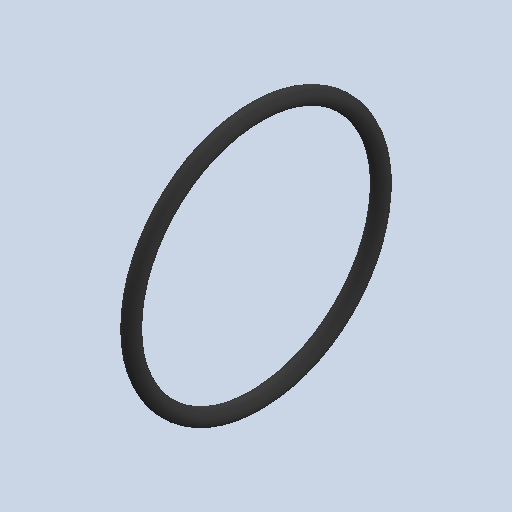
# Autodesk Inventor part: RD013_オーリング
Saved by Autodesk Inventor 2022 (Build 260153000, 153)
## iProperties
Created: 2021-10-14
Part Number: RD013_オーリング
Material: ゴム
Document SubType Name: Modeling
Designer: gilte
Density: 0.93 g/cm^3
Appearance: ゴム - 黒
Author: gilte
Autodesk Inventor part; units mm, degrees
ref_plane "YZ Plane" through (0, 0, 0) normal (1, 0, 0) x (0, 1, 0)
ref_plane "XZ Plane" through (0, 0, 0) normal (0, 1, 0) x (-1, 0, 0)
ref_plane "XY Plane" through (0, 0, 0) normal (0, 0, 1) x (1, 0, 0)
sketch "スケッチ1" plane through (0, 0, 0) normal (0, 0, 1) x (1, 0, 0)
  line L0 (0, 0) -> (5.9764, 0)
  line L1 (0, 0) -> (0, 24)
  circle A0 centre (0, 24) radius 1.5
  dimension "d0" = 24
  dimension "d1" = 3
  constraints: 4 end point, 1 centre point, 1 coincident, 1 horizontal, 1 vertical
  measures "d0" distance of L0.start L1.end
  measures "d1" diameter of A0
revolve "回転1" add sketch "スケッチ1" angle 360 about axis through (0, 0, 0) along (1, 0, 0)
